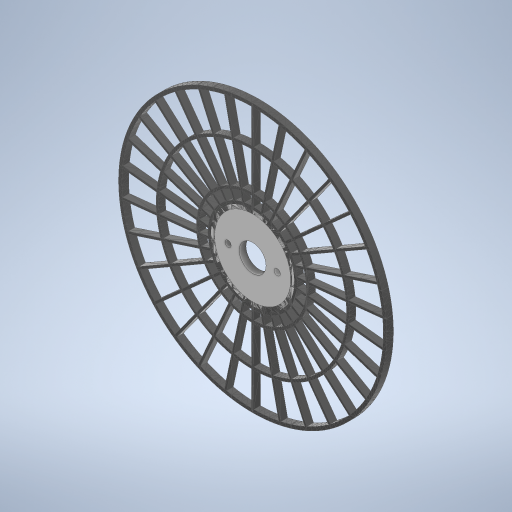
# Autodesk Inventor part: protection_cover_back
Saved by Autodesk Inventor 2024 (Build 280153000, 153)
## iProperties
Created: 2025-03-10
Part Number: protection_cover_back
Material: Generic
Document SubType Name: Modeling
Designer: 5454s
Density: 1 g/cm^3
Appearance: Default
Author: 5454s
Autodesk Inventor part; units mm, degrees
ref_plane "YZ Plane" through (0, 0, 0) normal (1, 0, 0) x (0, 1, 0)
ref_plane "XZ Plane" through (0, 0, 0) normal (0, 1, 0) x (-1, 0, 0)
ref_plane "XY Plane" through (0, 0, 0) normal (0, 0, 1) x (1, 0, 0)
sketch "Sketch1" plane through (36.808, 69.8575, 0) normal (0, 0, -1) x (-1, 0, 0)
  circle A0 centre (-23.1927, -9.8574) radius 18.7322
  circle A1 centre (-23.1927, -9.8574) radius 17.0007
  point P0 (36.808, -69.8575)
  constraints: 2 centre point, 1 coincident
extrude "Extrusion1" add sketch "Sketch1" against normal blind 3 contours A0 | A1
sketch "Sketch2" plane through (60.0007, 60.0001, 0) normal (0, 0, -1) x (-1, 0, 0)
  circle A0 centre (0, 0) radius 18.7322 projected
  circle A1 centre (0, 0) radius 16
  circle A2 centre (0, 0) radius 6
  circle A3 centre (-11, 0) radius 1.375
  circle A4 centre (11, 0) radius 1.375
  line L0 (0, 16) -> (0, -16)
  point P0 (60.0007, -60.0001)
  dimension "d2" = 32
  dimension "d3" = 12
  dimension "d4" = 2.75
  dimension "d5" = 22
  constraints: 4 centre point, 2 coincident, 2 end point, 2 point on circle, 1 equal radius, 1 symmetric about line, 1 vertical
  measures "d2" diameter of A1
  measures "d3" diameter of A2
  measures "d4" diameter of A4
  measures "d5" distance of A4.centre A3.centre
extrude "Extrusion2" cut sketch "Sketch2" against normal blind 3 contours L0 A2 | A2 L0 | A3 | A4
body "Solid1"
